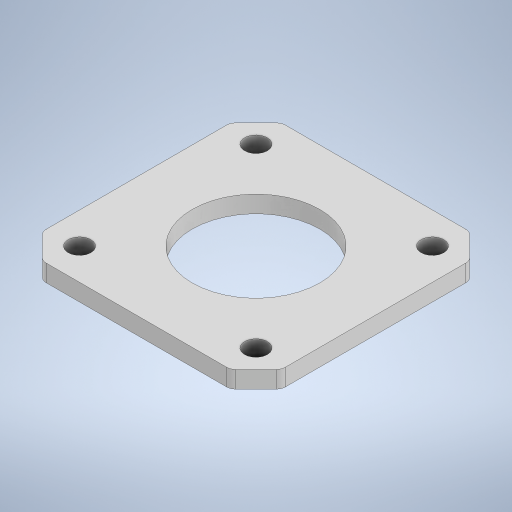
# Autodesk Inventor part: Part2
Saved by Autodesk Inventor 2024 (Build 280153000, 153)
## iProperties
Created: 2024-01-06
Part Number: Part2
Material: Generic
Document SubType Name: Modeling
Designer: jebes windows
Density: 1 g/cm^3
Appearance: Default
Author: jebes windows
## iProperties of the stored document Part2_3DPrint.ipt
Created: 2024-01-06
Part Number: Part2_3DPrint
Material: Generic
Document SubType Name: Modeling
Designer: jebes windows
Density: 1 g/cm^3
Appearance: Default
Author: jebes windows
Autodesk Inventor part; units mm, degrees
ref_plane "YZ Plane" through (0, 0, 0) normal (1, 0, 0) x (0, 1, 0)
ref_plane "XZ Plane" through (0, 0, 0) normal (0, 1, 0) x (-1, 0, 0)
ref_plane "XY Plane" through (0, 0, 0) normal (0, 0, 1) x (1, 0, 0)
ref_plane "Work Plane1" through (0, 0, 0) normal (0, 0, 1) x (1, 0, 0)
sketch "Sketch1" plane through (0, 0, 0) normal (0, 0, 1) x (1, 0, 0)
  arc A0 (16.9393, 20.5607) -> (15.8787, 21) centre (15.8787, 19.5) ccw projected
  line L0 (15.8787, 21) -> (-15.8787, 21) projected
  arc A1 (-15.8787, 21) -> (-16.9393, 20.5607) centre (-15.8787, 19.5) ccw projected
  line L1 (-16.9393, 20.5607) -> (-20.5607, 16.9393) projected
  arc A2 (-20.5607, 16.9393) -> (-21, 15.8787) centre (-19.5, 15.8787) ccw projected
  line L2 (-21, 15.8787) -> (-21, -15.8787) projected
  arc A3 (-21, -15.8787) -> (-20.5607, -16.9393) centre (-19.5, -15.8787) ccw projected
  line L3 (-20.5607, -16.9393) -> (-16.9393, -20.5607) projected
  arc A4 (-16.9393, -20.5607) -> (-15.8787, -21) centre (-15.8787, -19.5) ccw projected
  line L4 (-15.8787, -21) -> (15.8787, -21) projected
  arc A5 (15.8787, -21) -> (16.9393, -20.5607) centre (15.8787, -19.5) ccw projected
  line L5 (16.9393, -20.5607) -> (20.5607, -16.9393) projected
  arc A6 (20.5607, -16.9393) -> (21, -15.8787) centre (19.5, -15.8787) ccw projected
  line L6 (21, -15.8787) -> (21, 15.8787) projected
  arc A7 (21, 15.8787) -> (20.5607, 16.9393) centre (19.5, 15.8787) ccw projected
  line L7 (20.5607, 16.9393) -> (16.9393, 20.5607) projected
  circle A8 centre (-15.5, -15.5) radius 1.5 projected
  circle A9 centre (-15.5, 15.5) radius 1.5 projected
  circle A10 centre (15.5, -15.5) radius 1.5 projected
  circle A11 centre (15.5, 15.5) radius 1.5 projected
  circle A12 centre (0, 0) radius 11.2 projected
  circle A13 centre (-15.5, 15.5) radius 2
  circle A14 centre (-15.5, -15.5) radius 2
  circle A15 centre (15.5, -15.5) radius 2
  circle A16 centre (15.5, 15.5) radius 2
  point P0 (0, 0)
  dimension "d0" = 4
  dimension "d1" = 4
  dimension "d2" = 4
  dimension "d3" = 4
  constraints: 4 centre point, 4 coincident
  measures "d0" diameter of A13
  measures "d1" diameter of A14
  measures "d2" diameter of A15
  measures "d3" diameter of A16
extrude "Extrusion1" add sketch "Sketch1" along normal blind 3 contours L7 A7 L6 A6 L5 A5 L4 A4 L3 A3 L2 A2 L1 A1 L0 A0
body "Solid1"
